Autodesk Inventor part; units mm, degrees
(part 2 of 2)
  line L816 (2661.3236, 3996.6132) -> (2661.3236, 3742.6132)
  line L817 (2661.3236, 4022.0132) -> (2915.3236, 4022.0132)
  line L818 (2915.3236, 4022.0132) -> (2915.3236, 4276.0132)
  line L819 (2915.3236, 4276.0132) -> (2661.3236, 4276.0132)
  line L820 (2661.3236, 4276.0132) -> (2661.3236, 4022.0132)
  line L821 (2661.3236, 4301.4132) -> (2915.3236, 4301.4132)
  line L822 (2915.3236, 4301.4132) -> (2915.3236, 4555.4132)
  line L823 (2915.3236, 4555.4132) -> (2661.3236, 4555.4132)
  line L824 (2661.3236, 4555.4132) -> (2661.3236, 4301.4132)
  line L825 (2661.3236, 4580.8132) -> (2915.3236, 4580.8132)
  line L826 (2915.3236, 4580.8132) -> (2915.3236, 4834.8132)
  line L827 (2915.3236, 4834.8132) -> (2661.3236, 4834.8132)
  line L828 (2661.3236, 4834.8132) -> (2661.3236, 4580.8132)
  line L829 (2661.3236, 4860.2132) -> (2915.3236, 4860.2132)
  line L830 (2915.3236, 4860.2132) -> (2915.3236, 5114.2132)
  line L831 (2915.3236, 5114.2132) -> (2661.3236, 5114.2132)
  line L832 (2661.3236, 5114.2132) -> (2661.3236, 4860.2132)
  line L833 (2661.3236, 5139.6132) -> (2915.3236, 5139.6132)
  line L834 (2915.3236, 5139.6132) -> (2915.3236, 5393.6132)
  line L835 (2915.3236, 5393.6132) -> (2661.3236, 5393.6132)
  line L836 (2661.3236, 5393.6132) -> (2661.3236, 5139.6132)
  line L837 (2661.3236, 5419.0132) -> (2915.3236, 5419.0132)
  line L838 (2915.3236, 5419.0132) -> (2915.3236, 5673.0132)
  line L839 (2915.3236, 5673.0132) -> (2661.3236, 5673.0132)
  line L840 (2661.3236, 5673.0132) -> (2661.3236, 5419.0132)
  line L841 (2661.3236, 5698.4132) -> (2915.3236, 5698.4132)
  line L842 (2915.3236, 5698.4132) -> (2915.3236, 5952.4132)
  line L843 (2915.3236, 5952.4132) -> (2661.3236, 5952.4132)
  line L844 (2661.3236, 5952.4132) -> (2661.3236, 5698.4132)
  point P0 (0, 0)
  point P1 (273.7236, 237.4132)
  dimension "d4" = 254
  dimension "d5" = 254
  dimension "d8" = 279.4
  dimension "d11" = 279.4
  constraints: 1688 end point, 3 horizontal, 2 midpoint, 2 parallel, 2 vertical, 1 perpendicular, 1 point on line, 1672 other
  measures "d4" distance of L2.end L1.end
  measures "d5" distance of L1.end L0.end
  measures "d8" distance of L0.start L9.start
  measures "d11" distance of L0.start L89.start
extrude "Extrusion2" cut sketch "Sketch2" against normal through all
body "Solid1"
